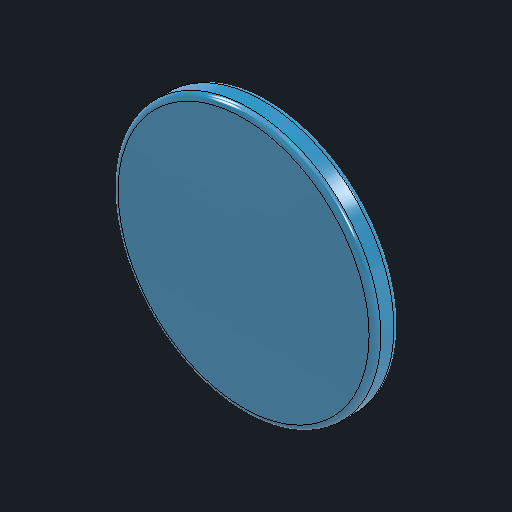
# Autodesk Inventor part: boron-under-mesh-plate
Saved by Autodesk Inventor 2026 (Build 300175050, 175E)
## iProperties
Created: 2024-12-16
Part Number: boron-under-mesh-plate
Material: Stainless Steel
Document SubType Name: Modeling
Designer: kuzmin
Density: 8 g/cm^3
Appearance: Sky Blue Dark
Author: kuzmin
Autodesk Inventor part; units mm, degrees
ref_plane "YZ Plane" through (0, 0, 0) normal (1, 0, 0) x (0, 1, 0)
ref_plane "XZ Plane" through (0, 0, 0) normal (0, 1, 0) x (-1, 0, 0)
ref_plane "XY Plane" through (0, 0, 0) normal (0, 0, 1) x (1, 0, 0)
sketch "Sketch1" plane through (0, 0, 0) normal (0, 0, 1) x (1, 0, 0)
  circle A0 centre (0, 0) radius 9
  dimension "d0" = 18
  constraints: 1 centre point, 1 coincident
  measures "d0" diameter of A0
extrude "Extrusion1" add sketch "Sketch1" along normal blind 1.7
fillet "Fillet1" radius 0.4 2 edges at (-9, 0, 1.7) (-9, 0, 0)
equation "\"d0\" = diameter"
equation "\"d1\" = thickness"
equation "\"thickness\" = 1.7"
equation "\"diameter\" = 18"
body "Solid1"
